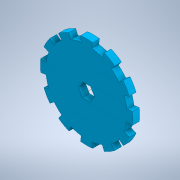
# Autodesk Inventor part: gearLock
Saved by Autodesk Inventor 2021.2 (Build 252289000, 289)
## iProperties
Created: 2020-11-07
Part Number: gearLock
Material: PC/ABS Plastic
Document SubType Name: Modeling
Designer: robst
Density: 0.357273 g/cm^3
Appearance: Sky Blue Medium
Author: robst
Autodesk Inventor part; units mm, degrees
ref_plane "YZ Plane" through (0, 0, 0) normal (1, 0, 0) x (0, 1, 0)
ref_plane "XZ Plane" through (0, 0, 0) normal (0, 1, 0) x (-1, 0, 0)
ref_plane "XY Plane" through (0, 0, 0) normal (0, 0, 1) x (1, 0, 0)
sketch "Sketch1" plane through (0, 0, 0) normal (0, 0, 1) x (1, 0, 0)
  circle A0 centre (0, 0) radius 38.1
  dimension "d0" = 76.2
  constraints: 1 centre point, 1 coincident
  measures "d0" diameter of A0
extrude "Extrusion1" add sketch "Sketch1" along normal mid plane 6.35
sketch "Sketch8" plane through (0, 0, 3.175) normal (0, 0, 1) x (1, 0, 0)
  arc A0 (5.624, 42.7187) -> (-5.624, 42.7187) centre (0, 0) ccw
  circle A1 centre (0, 0) radius 38.1 projected
  line L0 (4.973, 37.774) -> (5.624, 42.7187)
  line L1 (-4.973, 37.774) -> (-5.624, 42.7187)
  line L2 (0, 0) -> (0, 43.0873) construction
  arc A2 (4.973, 37.774) -> (-4.973, 37.774) centre (0, 0) ccw
  dimension "d40" = 4.9873
  dimension "d41" = 15
  dimension "d42" = 7.5
  constraints: 6 end point, 5 point on circle, 2 centre point, 2 coincident, 1 vertical
  measures "d40" radial gap between concentric circles of A1 A0
  measures "d41" angle of L0 L1
  measures "d42" angle of L1 L2
extrude "Extrusion9" add sketch "Sketch8" against normal blind 6.35 contours L0 A1 L1 A0
pattern_circular "Circular Pattern4" count 12 over 360 about axis through (0, 0, -10) along (0, 0, 1) of "Extrusion9"
sketch "Sketch10" plane through (0, 0, 3.175) normal (0, 0, 1) x (1, 0, 0)
  line L0 (7.3323, 0) -> (3.6662, -6.35)
  line L1 (3.6662, -6.35) -> (-3.6662, -6.35)
  line L2 (-3.6662, -6.35) -> (-7.3323, 0)
  line L3 (-7.3323, 0) -> (-3.6662, 6.35)
  line L4 (-3.6662, 6.35) -> (3.6662, 6.35)
  line L5 (3.6662, 6.35) -> (7.3323, 0)
  point P0 (0, 0)
  point P1 (0, 0)
  dimension "d55" = 12.7
  constraints: 12 end point, 1 coincident, 1 horizontal, 13 other
  measures "d55" distance between parallel lines of L1 L4
extrude "Extrusion11" cut sketch "Sketch10" against normal through all
equation "\"d0\" = externalDiameter"
equation "\"d40\" = depthOfExternalSpline"
equation "\"d55\" = hexSize"
equation "\"internalDiameter\" = 50.8"
equation "\"externalDiameter\" = 76.2"
equation "\"pi\" = 3.141593"
equation "\"depthOfInternalSpline\" = 0.5 * widthOfInternalSpline"
equation "\"depthOfExternalSpline\" = 0.5 * widthOfExternalSpline"
equation "\"thickness\" = 9.525"
equation "\"hexSize\" = 12.7"
equation "\"widthOfInternalSpline\" = 6.649704"
equation "\"widthOfExternalSpline\" = 9.974557"
body "Solid1"
